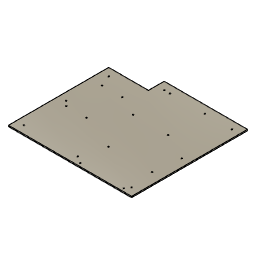
CIRAN1_Mounting_Plate (Autodesk Fusion 360 design; units mm, degrees)
Autodesk Fusion 360 part; units mm, degrees
sketch "Sketch1" plane through (0, 0, 0) normal (0, 0, 1) x (1, 0, 0)
  line L0 (102.9, 300) -> (102.9, 259.2)
  line L1 (318.5, 0) -> (0, 0)
  line L2 (102.9, 259.2) -> (0, 259.2)
  line L3 (318.5, 300) -> (102.9, 300)
  line L4 (318.5, 300) -> (318.5, 0)
  line L5 (0, 259.2) -> (0, 0)
  circle A0 centre (298.5, 280) radius 1.6
  circle A1 centre (122.9, 280) radius 1.6
  circle A2 centre (298.5, 20) radius 1.6
  circle A3 centre (20, 239.2) radius 1.6
  circle A4 centre (20, 20) radius 1.6
  circle A5 centre (20, 129.6) radius 1.6
  circle A6 centre (298.5, 150) radius 1.6
  circle A7 centre (159.25, 20) radius 1.6
  circle A8 centre (137.9, 280) radius 1.6
  line L6 (137.9, 280) -> (228.3, 280) construction
  circle A9 centre (228.3, 280) radius 1.6
  line L7 (137.9, 280) -> (137.9, 185) construction
  circle A10 centre (137.9, 185) radius 1.6
  line L8 (137.9, 185) -> (228.3, 185) construction
  circle A11 centre (228.3, 185) radius 1.6
  circle A12 centre (31.8301, 210) radius 1.6
  line L9 (31.8301, 210) -> (84.1301, 210) construction
  circle A13 centre (84.1301, 210) radius 1.6
  line L10 (31.8301, 210) -> (31.8301, 117.7) construction
  circle A14 centre (31.8301, 117.7) radius 1.6
  line L11 (84.1301, 210) -> (84.1301, 117.7) construction
  circle A15 centre (84.1301, 117.7) radius 1.6
  circle A16 centre (290.5, 8) radius 1.6
  line L12 (290.5, 8) -> (290.5, 81.2) construction
  circle A17 centre (290.5, 81.2) radius 1.6
  line L13 (290.5, 8) -> (177.6, 8) construction
  circle A18 centre (177.6, 8) radius 1.6
  line L14 (177.6, 8) -> (177.6, 81.2) construction
  circle A19 centre (177.6, 81.2) radius 1.6
  dimension "d3" = 318.5
  dimension "d4" = 300
  dimension "d5" = 40.8
  dimension "d6" = 102.9
  dimension "d9" = 3.2
  dimension "d10" = 20
  dimension "d11" = 20
  dimension "d12" = 3.2
  dimension "d13" = 20
  dimension "d14" = 20
  dimension "d15" = 3.2
  dimension "d16" = 20
  dimension "d17" = 20
  dimension "d18" = 3.2
  dimension "d19" = 20
  dimension "d20" = 20
  dimension "d21" = 3.2
  dimension "d22" = 20
  dimension "d23" = 20
  dimension "d24" = 3.2
  dimension "d25" = 20
  dimension "d26" = 109.6
  dimension "d27" = 3.2
  dimension "d28" = 20
  dimension "d29" = 130
  dimension "d30" = 3.2
  dimension "d31" = 20
  dimension "d32" = 159.25
  dimension "d33" = 3.2
  dimension "d36" = 90.4
  dimension "d37" = 3.2
  dimension "d38" = 95
  dimension "d39" = 3.2
  dimension "d40" = 90.4
  dimension "d41" = 3.2
  dimension "d42" = 3.2
  dimension "d43" = 52.3
  dimension "d44" = 3.2
  dimension "d45" = 92.3
  dimension "d46" = 3.2
  dimension "d47" = 92.3
  dimension "d48" = 3.2
  dimension "d49" = 35
  dimension "d50" = 20
  dimension "d51" = 3.2
  dimension "d52" = 8
  dimension "d53" = 8
  dimension "d54" = 73.2
  dimension "d55" = 3.2
  dimension "d56" = 112.9
  dimension "d57" = 3.2
  dimension "d58" = 73.2
  dimension "d59" = 3.2
  constraint perpendicular L3 L4
  constraint perpendicular L0 L3
  constraint perpendicular L0 L2
  constraint perpendicular L2 L5
  constraint perpendicular L1 L4
  constraint coincident L1.end L5.end
  constraint vertical L5
  constraint coincident A8.centre L6.start
  constraint horizontal L6
  constraint coincident L6.end A9.centre
  constraint perpendicular L6 L7
  constraint coincident L7.end A10.centre
  constraint perpendicular L7 L8
  constraint coincident L8.end A11.centre
  constraint coincident A12.centre L9.start
  constraint horizontal L9
  constraint coincident L9.end A13.centre
  constraint perpendicular L9 L10
  constraint coincident L10.end A14.centre
  constraint perpendicular L9 L11
  constraint coincident L11.end A15.centre
  constraint coincident A16.centre L12.start
  constraint vertical L12
  constraint coincident L12.end A17.centre
  constraint perpendicular L12 L13
  constraint coincident L13.end A18.centre
  constraint perpendicular L13 L14
  constraint coincident L14.end A19.centre
  measures "d3" distance of L4 L5
  measures "d4" distance of L1 L3
  measures "d5" distance of L0.end L0.start
  measures "d6" distance of L0.end L2.end
  measures "d9" diameter of A0
  measures "d10" distance of L3 A0.centre
  measures "d11" distance of L4 A0.centre
  measures "d12" diameter of A1
  measures "d13" distance of L3 A1.centre
  measures "d14" distance of L0 A1.centre
  measures "d15" diameter of A2
  measures "d16" distance of L4 A2.centre
  measures "d17" distance of L1 A2.centre
  measures "d18" diameter of A3
  measures "d19" distance of L5 A3.centre
  measures "d20" distance of L2 A3.centre
  measures "d21" diameter of A4
  measures "d22" distance of L5 A4.centre
  measures "d23" distance of L1 A4.centre
  measures "d24" diameter of A5
  measures "d25" distance of L5 A5.centre
  measures "d26" distance of A4.centre A5.centre
  measures "d27" diameter of A6
  measures "d28" distance of L4 A6.centre
  measures "d29" distance of A2.centre A6.centre
  measures "d30" diameter of A7
  measures "d31" distance of L1 A7.centre
  measures "d32" distance of L5 A7.centre
  measures "d33" diameter of A8
  measures "d36" distance of A8.centre L6.end
  measures "d37" diameter of A9
  measures "d38" distance of A8.centre L7.end
  measures "d39" diameter of A10
  measures "d40" distance of L7.end L8.end
  measures "d41" diameter of A11
  measures "d42" diameter of A12
  measures "d43" distance of A12.centre L9.end
  measures "d44" diameter of A13
  measures "d45" distance of A12.centre L10.end
  measures "d46" diameter of A14
  measures "d47" distance of L9.end L11.end
  measures "d48" diameter of A15
  measures "d49" distance of L0 A8.centre
  measures "d50" distance of L3 A8.centre
  measures "d51" diameter of A16
  measures "d52" horizontal distance of A2.centre A16.centre
  measures "d53" distance of L1 A16.centre
  measures "d54" distance of A16.centre L12.end
  measures "d55" diameter of A17
  measures "d56" distance of A16.centre L13.end
  measures "d57" diameter of A18
  measures "d58" distance of L13.end L14.end
  measures "d59" diameter of A19
extrude "Extrude1" add sketch "Sketch1" along normal blind 3
sketch "Mounting plate laser cut" plane through (0, 0, 3) normal (0, 0, 1) x (-1, 0, 0)
  circle A0 centre (-20, -129.6) radius 1.6
  circle A1 centre (-298.5, -280) radius 1.6
  circle A2 centre (-298.5, -20) radius 1.6
  circle A3 centre (-159.25, -20) radius 1.6
  circle A4 centre (-137.9, -280) radius 1.6
  circle A5 centre (-228.3, -280) radius 1.6
  circle A6 centre (-298.5, -150) radius 1.6
  circle A7 centre (-137.9, -185) radius 1.6
  circle A8 centre (-177.6, -8) radius 1.6
  circle A9 centre (-20, -239.2) radius 1.6
  circle A10 centre (-290.5, -8) radius 1.6
  circle A11 centre (-228.3, -185) radius 1.6
  circle A12 centre (-177.6, -81.2) radius 1.6
  circle A13 centre (-31.8301, -117.7) radius 1.6
  circle A14 centre (-290.5, -81.2) radius 1.6
  circle A15 centre (-84.1301, -117.7) radius 1.6
  circle A16 centre (-122.9, -280) radius 1.6
  circle A17 centre (-31.8301, -210) radius 1.6
  circle A18 centre (-84.1301, -210) radius 1.6
  circle A19 centre (-20, -20) radius 1.6
  line L0 (-318.5, -300) -> (-102.9, -300)
  line L1 (-102.9, -300) -> (-102.9, -259.2)
  line L2 (-102.9, -259.2) -> (0, -259.2)
  line L3 (0, -259.2) -> (0, 0)
  line L4 (0, 0) -> (-318.5, 0)
  line L5 (-318.5, 0) -> (-318.5, -300)
equation "d26 = ( 219.2 / 2 ) * 1 mm"
equation "d29 = ( 260 / 2 ) * 1 mm"
equation "d32 = ( 318.5 / 2 ) * 1 mm"
